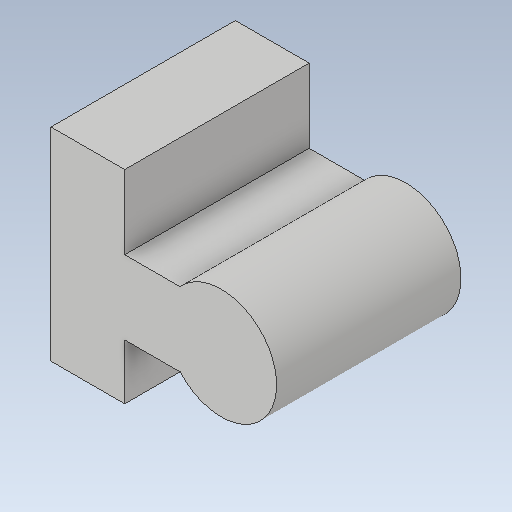
# Autodesk Inventor part: Hammer_Knautschzone
Saved by Autodesk Inventor 2021 (Build 250183000, 183)
## iProperties
Created: 2021-03-07
Part Number: Hammer_Knautschzone
Material: Generic
Document SubType Name: Modeling
Designer: Lukas
Density: 1 g/cm^3
Appearance: Default
Author: Lukas
Autodesk Inventor part; units mm, degrees
ref_plane "YZ Plane" through (0, 0, 0) normal (1, 0, 0) x (0, 1, 0)
ref_plane "XZ Plane" through (0, 0, 0) normal (0, 1, 0) x (-1, 0, 0)
ref_plane "XY Plane" through (0, 0, 0) normal (0, 0, 1) x (1, 0, 0)
sketch "Sketch1" plane through (0, 0, 0) normal (0, 0, 1) x (1, 0, 0)
  line L0 (-7, 5.5) -> (-7, -5.5)
  line L1 (-7, -5.5) -> (-3, -5.5)
  line L2 (-3, -5.5) -> (-3, -2.5)
  line L3 (-3, -2.5) -> (0, -2.5)
  line L4 (-7, 5.5) -> (-3, 5.5)
  line L5 (-3, 5.5) -> (-3, 1.5)
  line L6 (-3, 1.5) -> (0, 1.5)
  arc A0 (0, -2.5) -> (0, 1.5) centre (2.2361, -0.5) ccw
  point P0 (0, 0)
  point P1 (-7, 0)
  dimension "d0" = 3
  dimension "d1" = 4
  dimension "d2" = 2
  dimension "d3" = 3
  dimension "d4" = 4
  dimension "d8" = 4
  dimension "d9" = 3
  constraints: 14 end point, 5 perpendicular, 2 point on circle, 2 vertical alignment, 1 centre point, 1 horizontal, 1 horizontal alignment, 1 midpoint, 1 vertical
  measures "d0" radius of A0
  measures "d1" distance between parallel lines of L3 L6
  measures "d2" distance from line of A0.centre L6
  measures "d3" distance of L5.end L6.end
  measures "d4" distance of L0.start L4.end
  measures "d8" distance of L4.end L5.end
  measures "d9" distance of L1.end L2.end
extrude "Extrusion1" add sketch "Sketch1" along normal blind 10
equation "\"d2\" = 0.5 * d1"
body "Solid1"
